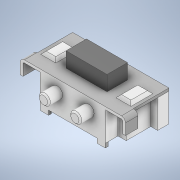
# Autodesk Inventor part: Button
Saved by Autodesk Inventor 2020 (Build 240168000, 168)
## iProperties
Created: 2022-02-24
Part Number: Button
Material: Типовые
Document SubType Name: Modeling
Designer: NoName
Density: 1 g/cm^3
Appearance: По умолчанию
Author: NoName
Autodesk Inventor part; units mm, degrees
ref_plane "YZ Plane" through (0, 0, 0) normal (1, 0, 0) x (0, 1, 0)
ref_plane "XZ Plane" through (0, 0, 0) normal (0, 1, 0) x (-1, 0, 0)
ref_plane "XY Plane" through (0, 0, 0) normal (0, 0, 1) x (1, 0, 0)
sketch "Эскиз2" plane through (0, 0, 0) normal (0, 1, 0) x (-1, 0, 0)
  line L0 (0, 0) -> (0, -3.5)
  line L1 (2.4, 0) -> (-2.4, 0)
  line L2 (-2.4, 0) -> (-2.4, -0.9)
  line L3 (-2.4, -0.9) -> (-3, -0.9)
  line L4 (-3, -0.9) -> (-3, -2.7)
  line L5 (-3, -2.7) -> (-3.5, -2.7)
  line L6 (-3.5, -2.7) -> (-3.5, -3.5)
  line L7 (-3.5, -3.5) -> (3.5, -3.5)
  line L8 (2.4, 0) -> (2.4, -0.9)
  line L9 (2.4, -0.9) -> (3, -0.9)
  line L10 (3, -0.9) -> (3, -2.7)
  line L11 (3, -2.7) -> (3.5, -2.7)
  line L12 (3.5, -2.7) -> (3.5, -3.5)
  dimension "d0" = 4.8
  dimension "d1" = 6
  dimension "d2" = 7
  dimension "d3" = 3.5
  dimension "d4" = 0.8
  dimension "d5" = 2.6
  constraints: 26 end point, 6 perpendicular, 4 symmetric about line, 2 midpoint, 1 horizontal, 1 vertical
  measures "d0" distance between parallel lines of L8 L2
  measures "d1" distance between parallel lines of L4 L10
  measures "d2" distance between parallel lines of L12 L6
  measures "d3" distance between parallel lines of L7 L1
  measures "d4" distance between parallel lines of L7 L5
  measures "d5" distance between parallel lines of L7 L3
extrude "Выдавливание1" add sketch "Эскиз2" along normal blind 2.1
sketch "Эскиз3" plane through (0, 2.1, 0) normal (0, 1, 0) x (1, 0, 0)
  line L0 (3.5, 2.7) -> (3.5, 3.5) projected
  line L1 (-2.4, 0) -> (2.4, 0) projected
  line L2 (-3.5, 3.5) -> (-3.5, 2.7) projected
  line L3 (3.5, 3.5) -> (-3.5, 3.5) projected
  line L4 (-3.525, 0.9) -> (-3.85, 0.9)
  line L5 (-3.85, 0.9) -> (-3.85, 0)
  line L6 (-3.85, 0) -> (3.85, 0)
  line L7 (3.85, 0) -> (3.85, 0.9)
  line L8 (3.85, 0.9) -> (3.525, 0.9)
  line L9 (-3.525, 0.9) -> (-3.525, 3.5057)
  line L10 (-3.525, 3.5057) -> (3.525, 3.5057)
  line L11 (3.525, 3.5057) -> (3.525, 0.9)
  point P0 (0, 0)
  point P1 (-2.4, 0)
  point P2 (2.4, 0)
  dimension "d8" = 7.7
  dimension "d9" = 0.9
  dimension "d33" = 7.05
  constraints: 16 end point, 3 point on line, 2 horizontal, 2 perpendicular, 2 vertical, 1 collinear, 1 midpoint
  measures "d8" distance of L5.end L6.end
  measures "d9" distance between parallel lines of L6 L8
  measures "d33" distance between parallel lines of L11 L9
extrude "Выдавливание2" add sketch "Эскиз3" along normal blind 0.2
sketch "Эскиз4" plane through (0, 2.1, 0) normal (0, -1, 0) x (1, 0, 0)
  line L0 (-3.85, 0) -> (3.85, 0) projected
  line L1 (-3.85, -0.9) -> (-3.65, -0.9)
  line L2 (-3.65, -0.9) -> (-3.65, 0)
  line L3 (-3.65, 0) -> (-3.85, 0)
  line L4 (-3.85, 0) -> (-3.85, -0.9)
  line L5 (0, -3.5) -> (0, 0)
  line L6 (-2.4, 0) -> (2.4, 0) projected
  line L7 (3.85, -0.9) -> (3.65, -0.9)
  line L8 (3.65, -0.9) -> (3.65, 0)
  line L9 (3.65, 0) -> (3.85, 0)
  line L10 (3.85, 0) -> (3.85, -0.9)
  point P0 (-3.85, -0.9)
  point P1 (3.85, 0)
  point P2 (3.85, 0)
  point P3 (3.65, 0)
  point P4 (-3.85, 0)
  dimension "d34" = 0.2
  constraints: 18 end point, 6 symmetric about line, 2 coincident, 2 parallel, 2 perpendicular, 1 horizontal, 1 point on line
  measures "d34" distance between parallel lines of L4 L2
extrude "Выдавливание3" add sketch "Эскиз4" along normal blind 0.9
fillet "Сопряжение1" radius 0.1 2 edges at (-3.65, 2.1, -0.45) (3.65, 2.1, -0.45)
fillet "Сопряжение1" radius 0.3 2 edges at (-3.85, 2.3, -0.45) (3.85, 2.3, -0.45)
sketch "Эскиз5" plane through (-2.4, 0, 0) normal (0, 0, 1) x (1, 0, 0)
  arc A0 (6.25, 2) -> (5.95, 2.3) centre (5.95, 2) ccw projected
  line L0 (-1.15, 2.3) -> (5.95, 2.3) projected
  arc A1 (-1.15, 2.3) -> (-1.45, 2) centre (-1.15, 2) ccw projected
  line L1 (-1.45, 1.2) -> (-1.45, 2) projected
  line L2 (-1.25, 1.2) -> (-1.45, 1.2) projected
  line L3 (-1.25, 2) -> (-1.25, 1.2) projected
  arc A2 (-1.15, 2.1) -> (-1.25, 2) centre (-1.15, 2) ccw projected
  line L4 (-1.15, 2.1) -> (0, 2.1) projected
  line L5 (0, 0) -> (0, 2.1) projected
  line L6 (0, 0) -> (4.8, 0) projected
  line L7 (4.8, 0) -> (4.8, 2.1) projected
  line L8 (4.8, 2.1) -> (5.95, 2.1) projected
  arc A3 (6.05, 2) -> (5.95, 2.1) centre (5.95, 2) ccw projected
  line L9 (6.05, 2) -> (6.05, 1.2) projected
  line L10 (6.25, 1.2) -> (6.05, 1.2) projected
  line L11 (6.25, 1.2) -> (6.25, 2) projected
  line L12 (2.4, 0) -> (2.4, 2.3)
  line L13 (-1.15, 2.3) -> (5.95, 2.3) projected
  line L14 (0, 0) -> (4.8, 0) projected
  line L15 (0.025, 0) -> (0.625, 0)
  line L16 (0.625, 0) -> (0.625, -0.3282)
  line L17 (0.625, -0.3282) -> (0.025, -0.3282)
  line L18 (0.025, -0.3282) -> (0.025, 0)
  line L19 (4.8, 0) -> (0, 0)
  line L20 (4.8, 0) -> (0, 0)
  line L21 (4.775, 0) -> (4.175, 0)
  line L22 (4.175, 0) -> (4.175, -0.3282)
  line L23 (4.175, -0.3282) -> (4.775, -0.3282)
  line L24 (4.775, -0.3282) -> (4.775, 0)
  point P0 (4.475, -0.3282)
  point P1 (0.325, -0.3282)
  dimension "d35" = 0.6
  dimension "d36" = 4.15
  constraints: 22 end point, 6 symmetric about line, 3 midpoint, 2 parallel, 2 point on line, 1 horizontal, 1 perpendicular
  measures "d35" distance between parallel lines of L22 L24
  measures "d36" distance of point (4.475, -0.328) point (0.325, -0.328)
extrude "Выдавливание4" add sketch "Эскиз5" against normal blind 0.2 contours L16 L17 L18 L6 | L6 L24 L23 L22
sketch "Эскиз6" plane through (0, 2.3, 0) normal (0, 1, 0) x (1, 0, 0)
  line L0 (-1.5, 1) -> (1.5, 1)
  line L1 (1.5, 1) -> (1.5, 2.5)
  line L2 (1.5, 2.5) -> (-1.5, 2.5)
  line L3 (-1.5, 2.5) -> (-1.5, 1)
  line L4 (-3.55, 0) -> (3.55, 0) projected
  point P0 (0, 0)
  point P1 (0, 1)
  point P2 (0, 0)
  point P3 (1.5, 1.75)
  dimension "d22" = 3
  dimension "d37" = 1.5
  dimension "d38" = 1
  constraints: 8 end point, 3 midpoint, 2 parallel, 1 horizontal, 1 perpendicular, 1 vertical alignment
  measures "d22" distance between parallel lines of L1 L3
  measures "d37" distance between parallel lines of L0 L2
  measures "d38" distance between parallel lines of L4 L0
extrude "Выдавливание5" add sketch "Эскиз6" along normal blind 1.1
sketch "Эскиз7" plane through (0, 2.3, 0) normal (0, 1, 0) x (1, 0, 0)
  line L0 (-3.3, 0.95) -> (-2.2, 0.95)
  line L1 (-2.2, 0.95) -> (-2.2, 2.55)
  line L2 (-2.2, 2.55) -> (-3.3, 2.55)
  line L3 (-3.3, 2.55) -> (-3.3, 0.95)
  line L4 (3.5, 3.5) -> (-3.5, 3.5) projected
  line L5 (0, 3.5) -> (0, 0)
  line L6 (3.3, 0.95) -> (2.2, 0.95)
  line L7 (2.2, 0.95) -> (2.2, 2.55)
  line L8 (2.2, 2.55) -> (3.3, 2.55)
  line L9 (3.3, 2.55) -> (3.3, 0.95)
  line L10 (-3.55, 0) -> (3.55, 0) projected
  point P0 (-3.3, 1.75)
  point P1 (-3.5, 1.75)
  point P2 (3.3, 1.75)
  dimension "d25" = 1.6
  dimension "d26" = 1.1
  dimension "d27" = 6.6
  dimension "d39" = 0.95
  constraints: 18 end point, 5 symmetric about line, 2 midpoint, 2 parallel, 1 horizontal, 1 horizontal alignment, 1 perpendicular, 1 vertical
  measures "d25" distance between parallel lines of L2 L0
  measures "d26" distance between parallel lines of L1 L3
  measures "d27" distance between parallel lines of L9 L3
  measures "d39" distance between parallel lines of L10 L0
extrude "Выдавливание6" add sketch "Эскиз7" along normal blind 0.2
chamfer "Фаска1" distance 0.2 angle 45 8 edges at (-2.75, 2.5, -2.55) (-2.2, 2.5, -1.75) (-2.75, 2.5, -0.95) (-3.3, 2.5, -1.75) (2.2, 2.5, -1.75) (2.75, 2.5, -2.55) (3.3, 2.5, -1.75) (2.75, 2.5, -0.95)
sketch "Эскиз8" plane through (-2.4, 0, 0) normal (0, 0, 1) x (1, 0, 0)
  circle A0 centre (3.55, 1.45) radius 0.4
  circle A1 centre (1.25, 1.45) radius 0.4
  line L0 (0.9, 2.3) -> (3.9, 2.3) projected
  line L1 (2.4, 2.3) -> (2.4, 0)
  line L2 (0.9, 3.4) -> (3.9, 3.4) projected
  dimension "d40" = 2.3
  dimension "d41" = 0.8
  dimension "d47" = 1.95
  constraints: 2 centre point, 2 end point, 1 midpoint, 1 vertical, 1 other
  measures "d40" distance of A1.centre A0.centre
  measures "d41" diameter of A1
  measures "d47" distance from line of L2 A1.centre
extrude "Выдавливание7" add sketch "Эскиз8" along normal blind 1
chamfer "Фаска2" distance 0.1 angle 45 2 edges at (0.75, 1.45, 1) (-1.55, 1.45, 1)
